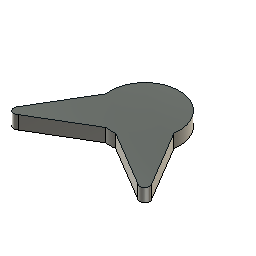
recirc_cell_valve_v2 v14 (Autodesk Fusion 360 archive; units mm, degrees)
design "Pinch Piece"
Autodesk Fusion 360 part; units mm, degrees
sketch "Sketch1" plane through (0, 0, 0) normal (0, 0, 1) x (1, 0, 0)
  line L0 (0, 0) -> (12.9082, -12.9082)
  line L1 (1.75, 0) -> (22.5, 0)
  line L2 (0, 0) -> (-12.9082, -12.9082)
  circle A0 centre (-12.2276, -12.2276) radius 0.9625
  circle A1 centre (12.2276, -12.2276) radius 0.9625
  circle A2 centre (0, 0) radius 6.675
  line L3 (-13.701, -10.7542) -> (-10.5388, -13.9165) construction
  line L4 (-12.9082, -11.5471) -> (-6.607, -0.9502)
  line L5 (-11.5471, -12.9082) -> (-0.9502, -6.607)
  line L6 (0, 1.75) -> (0, 22.5)
  line L7 (12.9082, -11.5471) -> (6.607, -0.9502)
  line L8 (11.5471, -12.9082) -> (0.9502, -6.607)
  dimension "d1" = 18.255
  dimension "d2" = 45
  dimension "d4" = -90
  dimension "d5" = 1.925
  dimension "d6" = 1.925
  dimension "d7" = 13.35
  dimension "d8" = 8
  constraint coincident L0.start L2.start
  constraint coincident L2 A0.centre
  constraint coincident L2.end A0
  constraint coincident L0 A1.centre
  constraint coincident L0.end A1
  constraint coincident A0.centre L3
  constraint perpendicular L2 L3
  constraint coincident L3 L4.start
  constraint coincident A0 L4.start
  constraint coincident L3 L5.start
  constraint coincident A0 L5.start
  constraint symmetric L2 L4 L5
  constraint coincident A2 L5.end
  constraint coincident A2 L4.end
  constraint symmetric L4.start L6 L7.start
  constraint symmetric L4.end L6 L7.end
  constraint symmetric L5.start L6 L8.start
  constraint symmetric L5.end L6 L8.end
  measures "d1" distance of L0.start L0.end
  measures "d2" angle of L0 L1
  measures "d5" diameter of A0
  measures "d6" diameter of A1
  measures "d7" diameter of A2
  measures "d8" distance of L4.end L5.end
extrude "Extrude1" add sketch "Sketch1" along normal blind 2.58
sketch "Sketch2" plane through (0, 0, 2.58) normal (0, 0, 1) x (-1, 0, 0)
  line L0 (-12.9082, 11.5471) -> (-6.607, 0.9502)
  arc A0 (-6.607, 0.9502) -> (6.607, 0.9502) centre (0, 0) ccw
  line L1 (6.607, 0.9502) -> (12.9082, 11.5471)
  arc A1 (12.9082, 11.5471) -> (11.5471, 12.9082) centre (12.2276, 12.2276) ccw
  line L2 (11.5471, 12.9082) -> (0.9502, 6.607)
  arc A2 (0.9502, 6.607) -> (-0.9502, 6.607) centre (0, 0) ccw
  line L3 (-0.9502, 6.607) -> (-11.5471, 12.9082)
  arc A3 (-11.5471, 12.9082) -> (-12.9082, 11.5471) centre (-12.2276, 12.2276) ccw
